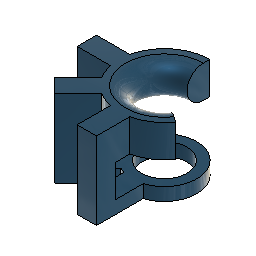
Design 18 v1 (Autodesk Fusion 360 design; units mm, degrees)
Autodesk Fusion 360 part; units mm, degrees
sketch "Sketch1" plane through (0, 0, 0) normal (1, 0, 0) x (0, 1, 0)
  line L0 (0, 25) -> (10, 25)
  line L1 (10, 25) -> (10, -25)
  line L2 (10, -25) -> (0, -25)
  arc A0 (0, 25) -> (0, -25) centre (0, 0) ccw
  line L3 (-60, 25) -> (-60, -25)
  dimension "d1" = 50
  dimension "d2" = 10
  dimension "d3" = 50
  dimension "d4" = 60
  constraint coincident A0.centre origin
  constraint horizontal L0
  constraint vertical L1
  constraint horizontal L2
  constraint vertical L3
  measures "d1" diameter of A0
  measures "d2" distance of L0.start L0.end
  measures "d3" distance of L0.start L2.end
  measures "d4" distance of A0.centre L3
revolve "Revolve1" add sketch "Sketch1" angle 235 about axis through (0, -60, 25) along (0, 0, 1) makes body 1
sketch "Sketch2" plane through (0, 0, 25) normal (0, 0, 1) x (-1, 0, 0)
  line L0 (0, 0) -> (0, -10)
  arc A0 (0, -10) -> (-57.3406, 100.1504) centre (0, 60) ccw
  line L1 (-57.3406, 100.1504) -> (-49.1491, 94.4146)
  arc A1 (0, 0) -> (-49.1491, 94.4146) centre (0, 60) ccw
  line L2 (62.0908, 75) -> (120, 75)
  line L3 (120, 75) -> (120, 45)
  line L4 (120, 45) -> (62.0908, 45)
  line L5 (62.0908, 45) -> (62.0908, 75)
  line L6 (120, 75) -> (90, 75)
  line L7 (90, 75) -> (90, 45)
  line L8 (90, 45) -> (120, 45)
  line L9 (120, 45) -> (120, 75)
  line L10 (74.2462, 155.4594) -> (95.4594, 134.2462)
  line L11 (54.5114, 93.2982) -> (33.2982, 114.5114)
  line L12 (33.2982, 114.5114) -> (74.2462, 155.4594)
  line L13 (95.4594, 134.2462) -> (54.5114, 93.2982)
  line L14 (53.033, 134.2462) -> (74.2462, 113.033)
  line L15 (-15, 180) -> (15, 180)
  line L16 (15, 122.0908) -> (-15, 122.0908)
  line L17 (-15, 122.0908) -> (-15, 180)
  line L18 (15, 180) -> (15, 122.0908)
  line L19 (-15, 150) -> (15, 150)
  dimension "d6" = 30
  dimension "d7" = 120
  dimension "d8" = 15
  dimension "d9" = 30
  dimension "d10" = 30
  dimension "d12" = 90
  constraint horizontal L2
  constraint vertical L3
  constraint horizontal L4
  constraint vertical L5
  constraint horizontal L6
  constraint vertical L7
  constraint horizontal L8
  constraint vertical L9
  measures "d6" distance of L2.start L4.end
  measures "d7" distance of A0.centre L3
  measures "d8" distance of A0.centre L4
  measures "d9" distance of L2.end L6.end
  measures "d10" distance of L2.end L3.end
extrude "Extrude1" add sketch "Sketch2" against normal blind 120 separate body contours L2 L3 L4 L6 L7 L8 L9 | L15 L17 L18 L19 | L10 L12 L13 L14 makes body 2 at (5, -150, -15) makes body 3 at (-60.1041, -127.1751, -15) makes body 4 at (-90, -65, -15)
extrude "Extrude2" add sketch "Sketch2" against normal blind 50 contours A0 L2 L4 L7 | A0 L17 L18 L19 | A0 L12 L13 L14 bodies 1 2 3 4
sketch "Sketch3" plane through (0, 0, -95) normal (0, 0, -1) x (1, 0, 0)
  line L0 (-53.033, 134.2462) -> (-74.2462, 155.4594)
  line L1 (-74.2462, 155.4594) -> (-95.4594, 134.2462)
  line L2 (-95.4594, 134.2462) -> (-74.2462, 113.033)
  line L3 (-74.2462, 113.033) -> (-53.033, 134.2462)
  line L4 (-15, 180) -> (-15, 128.374)
  line L5 (15, 180) -> (-15, 180)
  line L6 (15, 128.374) -> (15, 180)
  arc A0 (-15, 128.374) -> (-37.7411, 118.9543) centre (0, 60) ccw
  line L7 (-95.4594, 134.2462) -> (-58.9543, 97.7411)
  line L8 (-74.2462, 155.4594) -> (-95.4594, 134.2462)
  line L9 (-37.7411, 118.9543) -> (-74.2462, 155.4594)
  arc A1 (-58.9543, 97.7411) -> (-68.374, 75) centre (0, 60) ccw
  line L10 (-120, 75) -> (-68.374, 75)
  line L11 (-68.374, 45) -> (-120, 45)
  line L12 (-120, 45) -> (-120, 75)
  arc A2 (-68.374, 45) -> (0, -10) centre (0, 60) ccw
  line L13 (0, 0) -> (0, 25)
  line L14 (28.6703, 80.0752) -> (49.1491, 94.4146)
  arc A3 (57.3406, 100.1504) -> (15, 128.374) centre (0, 60) ccw
  line L15 (0, 0) -> (0, -10)
  line L16 (49.1491, 94.4146) -> (57.3406, 100.1504)
  arc A4 (28.6703, 80.0752) -> (0, 25) centre (0, 60) ccw
  circle A5 centre (0, 60) radius 35
  circle A6 centre (0, 60) radius 50
  line L17 (-15, 128.374) -> (15, 128.374)
  line L18 (15, 128.374) -> (15, 100.874)
  line L19 (15, 100.874) -> (-15, 100.874)
  line L20 (-15, 100.874) -> (-15, 128.374)
  line L21 (-39.5089, 78.2957) -> (-58.9543, 97.7411)
  line L22 (-58.9543, 97.7411) -> (-37.7411, 118.9543)
  line L23 (-18.2957, 99.5089) -> (-39.5089, 78.2957)
  line L24 (-37.7411, 118.9543) -> (-18.2957, 99.5089)
  line L25 (-40.874, 45) -> (-68.374, 45)
  line L26 (-68.374, 45) -> (-68.374, 75)
  line L27 (-40.874, 75) -> (-40.874, 45)
  line L28 (-68.374, 75) -> (-40.874, 75)
  dimension "d17" = 70
  dimension "d18" = 100
  dimension "d19" = 30
  dimension "d20" = 27.5
  dimension "d22" = 90
  constraint concentric A0 A5
  constraint concentric A5 A6
  constraint horizontal L17
  constraint vertical L18
  constraint horizontal L19
  constraint vertical L20
  constraint coincident L4.end A0.start
  measures "d17" diameter of A5
  measures "d18" diameter of A6
  measures "d19" distance of L4.end L6.start
  measures "d20" distance of L4.end L19.end
extrude "Extrude3" add sketch "Sketch3" against normal blind 20 contours L3 L7 L9 L22 | A6 L21 L22 L24 | L4 L5 L6 L17 | A6 L17 L18 L20 | A6 L21 L23 L24 | L13 L14 A4 A5 A6 L18 L19 L20 L21 L23 L24 L25 L27 L28 | L10 L11 L12 L26 | A6 L25 L26 L28 | A6 L18 L19 L20 | A6 L25 L27 L28 | L13 L14 A5 A6 bodies 1
